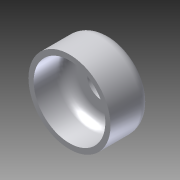
# Autodesk Inventor part: PVC Shooter Conveyor End Cap
Saved by Autodesk Inventor 2014 SP1 (Build 180222100, 222)
## iProperties
Created: 2012-03-04
Part Number: PVC Shooter Conveyor End Cap
Material: PVC-Piping
Document SubType Name: Modeling
Designer: Moses
Mass: 22.6203 g
Surface Area: 88.2985 cm^2
Volume: 16.1574 cm^3
Density: 1.4 g/cm^3
Appearance: Smooth - White
Author: Moses
Autodesk Inventor part; units mm, degrees
ref_plane "YZ Plane" through (0, 0, 0) normal (1, 0, 0) x (0, 1, 0)
ref_plane "XZ Plane" through (0, 0, 0) normal (0, 1, 0) x (-1, 0, 0)
ref_plane "XY Plane" through (0, 0, 0) normal (0, 0, 1) x (1, 0, 0)
sketch "Sketch1" plane through (0, 0, 0) normal (0, 0, 1) x (1, 0, 0)
  circle A0 centre (0, 0) radius 21.082
  circle A1 centre (0, 0) radius 24.13
  circle A2 centre (0, 0) radius 8.7313
  dimension "d0" = 42.164
  dimension "d1" = 48.26
  dimension "d8" = 17.4625
  constraints: 3 centre point, 3 coincident
  measures "d0" diameter of A0
  measures "d1" diameter of A1
  measures "d8" diameter of A2
extrude "Extrusion1" add sketch "Sketch1" along normal blind 19.05 contours A1
extrude "Extrusion2" add sketch "Sketch1" against normal blind 5.08 contours A0 | A1 | A2
fillet "Fillet1" radius 6.35 1 edges at (-24.13, 0, -5.08)
fillet "Fillet2" radius 6.35 1 edges at (-21.082, 0, 0)
extrude "Extrusion3" cut sketch "Sketch1" against normal blind 5.08 contours A2
body "Solid1"
